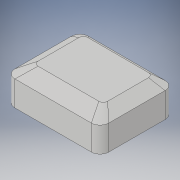
# Autodesk Inventor part: printer
Saved by Autodesk Inventor 2017 (Build 210142000, 142)
## iProperties
Created: 2018-04-03
Part Number: printer
Material: Generic
Document SubType Name: Modeling
Designer: Braxton
Density: 1 g/cm^3
Appearance: Default
Author: Braxton
Autodesk Inventor part; units mm, degrees
ref_plane "YZ Plane" through (0, 0, 0) normal (1, 0, 0) x (0, 1, 0)
ref_plane "XZ Plane" through (0, 0, 0) normal (0, 1, 0) x (-1, 0, 0)
ref_plane "XY Plane" through (0, 0, 0) normal (0, 0, 1) x (1, 0, 0)
sketch "Sketch1" plane through (0, 0, 0) normal (0, 1, 0) x (-1, 0, 0)
  line L0 (20.6375, 12.3693) -> (20.6375, -12.3693)
  line L1 (16.801, 16.2057) -> (0, 16.2057)
  line L2 (0, 0) -> (0, 16.2057) construction
  line L3 (16.801, -16.2057) -> (0, -16.2057)
  arc A0 (16.801, -16.2057) -> (20.6375, -12.3693) centre (16.801, -12.3693) ccw
  arc A1 (20.6375, 12.3693) -> (16.801, 16.2057) centre (16.801, 12.3693) ccw
  line L4 (20.6375, 0) -> (0, 0) construction
  line L5 (-20.6375, 12.3693) -> (-20.6375, -12.3693)
  line L6 (-16.801, 16.2057) -> (0, 16.2057)
  line L7 (-16.801, -16.2057) -> (0, -16.2057)
  arc A2 (-20.6375, -12.3693) -> (-16.801, -16.2057) centre (-16.801, -12.3693) ccw
  arc A3 (-16.801, 16.2057) -> (-20.6375, 12.3693) centre (-16.801, 12.3693) ccw
  line L8 (-20.6375, 0) -> (0, 0) construction
  dimension "d3" = 3.8365
  dimension "d4" = 32.4115
  dimension "d5" = 3.8365
  dimension "d6" = 20.6375
  constraints: 18 end point, 8 point on circle, 7 symmetric about line, 4 centre point, 4 tangent, 3 perpendicular, 1 coincident, 1 horizontal, 1 midpoint, 1 point on line, 2 other
  measures "d3" radius of A0
  measures "d4" distance between parallel lines of L1 L3
  measures "d5" radius of A1
  measures "d6" distance from line of L1.end L0
extrude "middle of body" add sketch "Sketch1" along normal blind 11.0384
ref_plane "top of printer" through (0, 14.2304, 0) normal (0, 1, 0) x (1, 0, 0)
sketch "Sketch2" plane through (0, 14.2304, 0) normal (0, 1, 0) x (1, 0, 0)
  line L0 (-13.3615, -9.4589) -> (0, -9.4589)
  line L1 (0, 12.3693) -> (-13.3615, 12.3693)
  line L2 (-15.2797, 10.451) -> (-15.2797, -7.5406)
  arc A0 (-15.2797, -7.5406) -> (-13.3615, -9.4589) centre (-13.3615, -7.5406) ccw
  arc A1 (-13.3615, 12.3693) -> (-15.2797, 10.451) centre (-13.3615, 10.451) ccw
  line L3 (0, -9.4589) -> (0, 0) construction
  line L4 (0, 0) -> (0, 12.3693) construction
  line L5 (16.801, 16.2057) -> (-16.801, 16.2057) projected
  line L6 (13.3615, -9.4589) -> (0, -9.4589)
  line L7 (0, 12.3693) -> (13.3615, 12.3693)
  line L8 (15.2797, 10.451) -> (15.2797, -7.5406)
  arc A2 (13.3615, -9.4589) -> (15.2797, -7.5406) centre (13.3615, -7.5406) ccw
  arc A3 (15.2797, 10.451) -> (13.3615, 12.3693) centre (13.3615, 10.451) ccw
  dimension "d10" = 15.2797
  dimension "d11" = 21.8281
  dimension "d12" = 3.8365
  dimension "d13" = 1.9182
  constraints: 16 end point, 8 point on circle, 6 symmetric about line, 4 centre point, 4 tangent, 2 perpendicular, 1 coincident, 1 collinear, 1 equal radius, 2 other
  measures "d10" distance from line of L1.start L2
  measures "d11" distance between parallel lines of L0 L1
  measures "d12" distance between parallel lines of L5 L1
  measures "d13" radius of A1
loft "top part of printer" add profiles "Sketch2" section 1 edges at (8.4005, 11.0384, 16.2057) (-8.4005, 11.0384, 16.2057) (19.5138, 11.0384, 15.0821) (20.6375, 11.0384, 0) (19.5138, 11.0384, -15.0821) (-8.4005, 11.0384, -16.2057) (8.4005, 11.0384, -16.2057) (-19.5138, 11.0384, -15.0821) (-20.6375, 11.0384, 0) (-19.5138, 11.0384, 15.0821)
sketch "Sketch39" plane through (-16.801, 11.0384, 16.2057) normal (0, 0.9039427, 0.4276535) x (1, 0, 0)
  circle A0 centre (3.4396, 5.0371) radius 0.4043
  line L0 (3.8689, 2.2071) -> (4.0551, 2.2071)
  line L1 (4.0551, 2.2071) -> (4.0551, 2.0209)
  line L2 (4.0551, 2.0209) -> (3.8689, 2.0209)
  line L3 (3.8688, 2.0209) -> (3.8688, 2.2071)
  arc A1 (3.8689, 2.2071) -> (3.8688, 2.2071) centre (3.8689, 2.2071) ccw
  arc A2 (3.8688, 2.0209) -> (3.8689, 2.0209) centre (3.8689, 2.0209) ccw
  line L4 (3.962, 2.2071) -> (3.962, 2.0209)
  arc A3 (4.0551, 2.2071) -> (4.0551, 2.2071) centre (4.0551, 2.2071) ccw
  arc A4 (4.0551, 2.0209) -> (4.0551, 2.0209) centre (4.0551, 2.0209) ccw
  line L5 (4.0551, 2.2632) -> (3.8689, 2.2632)
  arc A5 (3.8689, 2.2632) -> (3.8128, 2.2071) centre (3.8689, 2.2071) ccw
  line L6 (3.8128, 2.2071) -> (3.8128, 2.0209)
  arc A6 (3.8128, 2.0209) -> (3.8689, 1.9648) centre (3.8689, 2.0209) ccw
  line L7 (3.8689, 1.9648) -> (4.0551, 1.9648)
  arc A7 (4.0551, 1.9648) -> (4.1112, 2.0209) centre (4.0551, 2.0209) ccw
  line L8 (4.1112, 2.0209) -> (4.1112, 2.2071)
  arc A8 (4.1112, 2.2071) -> (4.0551, 2.2632) centre (4.0551, 2.2071) ccw
  circle A9 centre (3.4396, 5.0371) radius 0.4604
  arc A10 (5.1922, 4.9492) -> (4.8493, 4.6063) centre (5.1922, 4.6063) ccw
  arc A11 (4.8493, 1.9753) -> (5.1922, 1.6324) centre (5.1922, 1.9753) ccw
  line L9 (6.5077, 5.735) -> (6.5077, 2.5728) construction
  arc A12 (8.1661, 4.6063) -> (7.8232, 4.9492) centre (7.8232, 4.6063) ccw
  arc A13 (7.8232, 1.6324) -> (8.1661, 1.9753) centre (7.8232, 1.9753) ccw
  line L10 (7.8232, 5.0053) -> (5.1922, 5.0053)
  arc A14 (5.1922, 5.0053) -> (4.7932, 4.6063) centre (5.1922, 4.6063) ccw
  line L11 (4.7932, 4.6063) -> (4.7932, 1.9753)
  arc A15 (4.7932, 1.9753) -> (5.1922, 1.5763) centre (5.1922, 1.9753) ccw
  line L12 (5.1922, 1.5763) -> (7.8232, 1.5763)
  arc A16 (7.8232, 1.5763) -> (8.2222, 1.9753) centre (7.8232, 1.9753) ccw
  line L13 (8.2222, 1.9753) -> (8.2222, 4.6063)
  arc A17 (8.2222, 4.6063) -> (7.8232, 5.0053) centre (7.8232, 4.6063) ccw
  arc A18 (10.4923, 5.9298) -> (10.215, 5.6525) centre (10.4923, 5.6525) ccw
  line L14 (17.5445, 6.4989) -> (17.5445, 1.1088) construction
  arc A19 (10.215, 0.9292) -> (10.4923, 0.6519) centre (10.4923, 0.9292) ccw
  arc A20 (24.874, 5.6525) -> (24.5967, 5.9298) centre (24.5967, 5.6525) ccw
  arc A21 (24.5967, 0.6519) -> (24.874, 0.9292) centre (24.5967, 0.9292) ccw
  line L15 (24.5967, 5.9859) -> (10.4923, 5.9859)
  arc A22 (10.4923, 5.9859) -> (10.1589, 5.6525) centre (10.4923, 5.6525) ccw
  line L16 (10.1589, 5.6525) -> (10.1589, 0.9292)
  arc A23 (10.1589, 0.9292) -> (10.4923, 0.5958) centre (10.4923, 0.9292) ccw
  line L17 (10.4923, 0.5958) -> (24.5967, 0.5958)
  arc A24 (24.5967, 0.5958) -> (24.9301, 0.9292) centre (24.5967, 0.9292) ccw
  arc A25 (24.9301, 5.6525) -> (24.5967, 5.9859) centre (24.5967, 5.6525) ccw
  line L18 (10.8682, 5.5287) -> (15.7881, 5.5287)
  line L19 (15.8708, 5.446) -> (15.8708, 1.7707)
  line L20 (15.7881, 1.688) -> (10.8682, 1.688)
  line L21 (10.7855, 1.7707) -> (10.7855, 5.446)
  arc A26 (10.8682, 5.5287) -> (10.7855, 5.446) centre (10.8682, 5.446) ccw
  arc A27 (10.7855, 1.7707) -> (10.8682, 1.688) centre (10.8682, 1.7707) ccw
  line L22 (13.3281, 5.5287) -> (13.3281, 1.688) construction
  arc A28 (15.8708, 5.446) -> (15.7881, 5.5287) centre (15.7881, 5.446) ccw
  arc A29 (15.7881, 1.688) -> (15.8708, 1.7707) centre (15.7881, 1.7707) ccw
  line L23 (15.7881, 5.5848) -> (10.8682, 5.5848)
  arc A30 (10.8682, 5.5848) -> (10.7294, 5.446) centre (10.8682, 5.446) ccw
  line L24 (10.7294, 5.446) -> (10.7294, 1.7707)
  arc A31 (10.7294, 1.7707) -> (10.8682, 1.6319) centre (10.8682, 1.7707) ccw
  line L25 (10.8682, 1.6319) -> (15.7881, 1.6319)
  arc A32 (15.7881, 1.6319) -> (15.9269, 1.7707) centre (15.7881, 1.7707) ccw
  line L26 (15.9269, 1.7707) -> (15.9269, 5.446)
  arc A33 (15.9269, 5.446) -> (15.7881, 5.5848) centre (15.7881, 5.446) ccw
  line L27 (10.7855, 0.6519) -> (10.7855, 1.1451)
  arc A34 (10.8733, 1.2329) -> (10.7855, 1.1451) centre (10.8733, 1.1451) ccw
  arc A35 (10.8733, 1.289) -> (10.7294, 1.1451) centre (10.8733, 1.1451) ccw
  line L28 (10.7294, 1.1451) -> (10.7294, 0.6519)
  line L29 (15.8708, 1.1451) -> (15.8708, 0.6519)
  arc A36 (15.8708, 1.1451) -> (15.7829, 1.2329) centre (15.7829, 1.1451) ccw
  line L30 (15.9269, 0.6519) -> (15.9269, 1.1451)
  arc A37 (15.9269, 1.1451) -> (15.7829, 1.289) centre (15.7829, 1.1451) ccw
  line L31 (16.4973, 5.9298) -> (18.5494, 5.9298)
  line L32 (18.5494, 5.9298) -> (18.5494, 4.6524)
  line L33 (18.5494, 4.6524) -> (16.4973, 4.6524)
  line L34 (16.4973, 4.6524) -> (16.4973, 5.9298)
  line L35 (16.4973, 4.5963) -> (18.5494, 4.5963)
  line L36 (18.5494, 4.5963) -> (18.5494, 3.3189)
  line L37 (18.5494, 3.3189) -> (16.4973, 3.3189)
  line L38 (16.4973, 3.3189) -> (16.4973, 4.5963)
  line L39 (16.4973, 3.2628) -> (18.5494, 3.2628)
  line L40 (18.5494, 3.2628) -> (18.5494, 1.9854)
  line L41 (18.5494, 1.9854) -> (16.4973, 1.9854)
  line L42 (16.4973, 1.9854) -> (16.4973, 3.2628)
  line L43 (16.4973, 1.9293) -> (18.5494, 1.9293)
  line L44 (18.5494, 1.9293) -> (18.5494, 0.6519)
  line L45 (18.5494, 0.6519) -> (16.4973, 0.6519)
  line L46 (16.4973, 0.6519) -> (16.4973, 1.9293)
  line L47 (18.6055, 5.9298) -> (20.6576, 5.9298)
  line L48 (20.6576, 5.9298) -> (20.6576, 4.6524)
  line L49 (20.6576, 4.6524) -> (18.6055, 4.6524)
  line L50 (18.6055, 4.6524) -> (18.6055, 5.9298)
  line L51 (18.6055, 4.5963) -> (20.6576, 4.5963)
  line L52 (20.6576, 4.5963) -> (20.6576, 3.3189)
  line L53 (20.6576, 3.3189) -> (18.6055, 3.3189)
  line L54 (18.6055, 3.3189) -> (18.6055, 4.5963)
  line L55 (18.6055, 3.2628) -> (20.6576, 3.2628)
  line L56 (20.6576, 3.2628) -> (20.6576, 1.9854)
  line L57 (20.6576, 1.9854) -> (18.6055, 1.9854)
  line L58 (18.6055, 1.9854) -> (18.6055, 3.2628)
  line L59 (18.6055, 1.9293) -> (20.6576, 1.9293)
  line L60 (20.6576, 1.9293) -> (20.6576, 0.6519)
  line L61 (20.6576, 0.6519) -> (18.6055, 0.6519)
  line L62 (18.6055, 0.6519) -> (18.6055, 1.9293)
  line L63 (20.7137, 5.9298) -> (22.7658, 5.9298)
  line L64 (22.7658, 5.9298) -> (22.7658, 4.6524)
  line L65 (22.7658, 4.6524) -> (20.7137, 4.6524)
  line L66 (20.7137, 4.6524) -> (20.7137, 5.9298)
  line L67 (20.7137, 4.5963) -> (22.7658, 4.5963)
  line L68 (22.7658, 4.5963) -> (22.7658, 3.3189)
  line L69 (22.7658, 3.3189) -> (20.7137, 3.3189)
  line L70 (20.7137, 3.3189) -> (20.7137, 4.5963)
  line L71 (20.7137, 3.2628) -> (22.7658, 3.2628)
  line L72 (22.7658, 3.2628) -> (22.7658, 1.9854)
  line L73 (22.7658, 1.9854) -> (20.7137, 1.9854)
  line L74 (20.7137, 1.9854) -> (20.7137, 3.2628)
  line L75 (20.7137, 1.9293) -> (22.7658, 1.9293)
  line L76 (22.7658, 1.9293) -> (22.7658, 0.6519)
  line L77 (22.7658, 0.6519) -> (20.7137, 0.6519)
  line L78 (20.7137, 0.6519) -> (20.7137, 1.9293)
  line L79 (24.874, 4.6524) -> (22.8219, 4.6524)
  line L80 (22.8219, 4.6524) -> (22.8219, 5.9298)
  line L81 (22.8219, 4.5963) -> (24.874, 4.5963)
  line L82 (24.874, 4.5963) -> (24.874, 3.3189)
  line L83 (24.874, 3.3189) -> (22.8219, 3.3189)
  line L84 (22.8219, 3.3189) -> (22.8219, 4.5963)
  line L85 (22.8219, 3.2628) -> (24.874, 3.2628)
  line L86 (24.874, 3.2628) -> (24.874, 1.9854)
  line L87 (24.874, 1.9854) -> (22.8219, 1.9854)
  line L88 (22.8219, 1.9854) -> (22.8219, 3.2628)
  line L89 (22.8219, 1.9293) -> (24.874, 1.9293)
  line L90 (22.8219, 0.6519) -> (22.8219, 1.9293)
  line L91 (25.7461, 5.6668) -> (26.4975, 5.6668)
  line L92 (26.4975, 5.6668) -> (26.4975, 4.9154)
  line L93 (26.4975, 4.9154) -> (25.7461, 4.9154)
  line L94 (25.7461, 4.9154) -> (25.7461, 5.6668)
  line L95 (26.1218, 5.6668) -> (26.1218, 4.9154) construction
  arc A38 (25.7461, 5.6668) -> (25.7461, 5.6668) centre (25.7461, 5.6668) ccw
  arc A39 (25.7461, 4.9154) -> (25.7461, 4.9154) centre (25.7461, 4.9154) ccw
  arc A40 (26.4975, 5.6668) -> (26.4975, 5.6668) centre (26.4975, 5.6668) ccw
  arc A41 (26.4975, 4.9154) -> (26.4975, 4.9154) centre (26.4975, 4.9154) ccw
  line L96 (26.4975, 5.7229) -> (25.7461, 5.7229)
  arc A42 (25.7461, 5.7229) -> (25.69, 5.6668) centre (25.7461, 5.6668) ccw
  line L97 (25.69, 5.6668) -> (25.69, 4.9154)
  arc A43 (25.69, 4.9154) -> (25.7461, 4.8593) centre (25.7461, 4.9154) ccw
  line L98 (25.7461, 4.8593) -> (26.4975, 4.8593)
  arc A44 (26.4975, 4.8593) -> (26.5536, 4.9154) centre (26.4975, 4.9154) ccw
  line L99 (26.5536, 4.9154) -> (26.5536, 5.6668)
  arc A45 (26.5536, 5.6668) -> (26.4975, 5.7229) centre (26.4975, 5.6668) ccw
  line L100 (25.7461, 1.9293) -> (26.4975, 1.9293)
  line L101 (26.4975, 1.9293) -> (26.4975, 1.1779)
  line L102 (26.4975, 1.1779) -> (25.7461, 1.1779)
  line L103 (25.7461, 1.1779) -> (25.7461, 1.9293)
  line L104 (26.1218, 1.9293) -> (26.1218, 1.1779) construction
  arc A46 (25.7461, 1.9293) -> (25.7461, 1.9293) centre (25.7461, 1.9293) ccw
  arc A47 (25.7461, 1.1779) -> (25.7461, 1.1779) centre (25.7461, 1.1779) ccw
  arc A48 (26.4975, 1.9293) -> (26.4975, 1.9293) centre (26.4975, 1.9293) ccw
  arc A49 (26.4975, 1.1779) -> (26.4975, 1.1779) centre (26.4975, 1.1779) ccw
  line L105 (26.4975, 1.9854) -> (25.7461, 1.9854)
  arc A50 (25.7461, 1.9854) -> (25.69, 1.9293) centre (25.7461, 1.9293) ccw
  line L106 (25.69, 1.9293) -> (25.69, 1.1779)
  arc A51 (25.69, 1.1779) -> (25.7461, 1.1218) centre (25.7461, 1.1779) ccw
  line L107 (25.7461, 1.1218) -> (26.4975, 1.1218)
  arc A52 (26.4975, 1.1218) -> (26.5536, 1.1779) centre (26.4975, 1.1779) ccw
  line L108 (26.5536, 1.1779) -> (26.5536, 1.9293)
  arc A53 (26.5536, 1.9293) -> (26.4975, 1.9854) centre (26.4975, 1.9293) ccw
  line L109 (25.7461, 3.6665) -> (26.4975, 3.6665)
  line L110 (26.4975, 3.6665) -> (26.4975, 2.9151)
  line L111 (26.4975, 2.9151) -> (25.7461, 2.9151)
  line L112 (25.7461, 2.9151) -> (25.7461, 3.6665)
  line L113 (26.1218, 3.6665) -> (26.1218, 2.9151) construction
  arc A54 (25.7461, 3.6665) -> (25.7461, 3.6665) centre (25.7461, 3.6665) ccw
  arc A55 (25.7461, 2.9151) -> (25.7461, 2.9151) centre (25.7461, 2.9151) ccw
  arc A56 (26.4975, 3.6665) -> (26.4975, 3.6665) centre (26.4975, 3.6665) ccw
  arc A57 (26.4975, 2.9151) -> (26.4975, 2.9151) centre (26.4975, 2.9151) ccw
  line L114 (26.4975, 3.7226) -> (25.7461, 3.7226)
  arc A58 (25.7461, 3.7226) -> (25.69, 3.6665) centre (25.7461, 3.6665) ccw
  line L115 (25.69, 3.6665) -> (25.69, 2.9151)
  arc A59 (25.69, 2.9151) -> (25.7461, 2.859) centre (25.7461, 2.9151) ccw
  line L116 (25.7461, 2.859) -> (26.4975, 2.859)
  arc A60 (26.4975, 2.859) -> (26.5536, 2.9151) centre (26.4975, 2.9151) ccw
  line L117 (26.5536, 2.9151) -> (26.5536, 3.6665)
  arc A61 (26.5536, 3.6665) -> (26.4975, 3.7226) centre (26.4975, 3.6665) ccw
  arc A62 (27.3029, 1.1779) -> (27.359, 1.1218) centre (27.359, 1.1779) ccw
  arc A63 (27.359, 1.1779) -> (27.359, 1.1779) centre (27.359, 1.1779) ccw
  arc A64 (28.9306, 1.1779) -> (28.9306, 1.1779) centre (28.9306, 1.1779) ccw
  arc A65 (28.9306, 1.1218) -> (28.9867, 1.1779) centre (28.9306, 1.1779) ccw
  line L118 (27.359, 1.1218) -> (28.9306, 1.1218)
  line L119 (28.9306, 1.1779) -> (27.359, 1.1779)
  line L120 (27.359, 1.1779) -> (27.359, 2.7495)
  line L121 (27.3029, 2.7495) -> (27.3029, 1.1779)
  arc A66 (27.359, 2.8056) -> (27.3029, 2.7495) centre (27.359, 2.7495) ccw
  arc A67 (27.359, 2.7495) -> (27.359, 2.7495) centre (27.359, 2.7495) ccw
  line L122 (28.1448, 2.7495) -> (28.1448, 1.1779) construction
  line L123 (28.9306, 2.7495) -> (28.9306, 1.1779)
  line L124 (28.9867, 1.1779) -> (28.9867, 2.7495)
  line L125 (27.359, 2.7495) -> (28.9306, 2.7495)
  line L126 (28.9306, 2.8056) -> (27.359, 2.8056)
  arc A68 (28.9306, 2.7495) -> (28.9306, 2.7495) centre (28.9306, 2.7495) ccw
  arc A69 (28.9867, 2.7495) -> (28.9306, 2.8056) centre (28.9306, 2.7495) ccw
  arc A70 (27.3029, 4.0952) -> (27.359, 4.0391) centre (27.359, 4.0952) ccw
  arc A71 (27.359, 4.0952) -> (27.359, 4.0952) centre (27.359, 4.0952) ccw
  arc A72 (28.9306, 4.0952) -> (28.9306, 4.0952) centre (28.9306, 4.0952) ccw
  arc A73 (28.9306, 4.0391) -> (28.9867, 4.0952) centre (28.9306, 4.0952) ccw
  line L127 (27.359, 4.0391) -> (28.9306, 4.0391)
  line L128 (28.9306, 4.0952) -> (27.359, 4.0952)
  line L129 (27.359, 4.0952) -> (27.359, 5.6668)
  line L130 (27.3029, 5.6668) -> (27.3029, 4.0952)
  arc A74 (27.359, 5.7229) -> (27.3029, 5.6668) centre (27.359, 5.6668) ccw
  arc A75 (27.359, 5.6668) -> (27.359, 5.6668) centre (27.359, 5.6668) ccw
  line L131 (28.1448, 5.6668) -> (28.1448, 4.0952) construction
  line L132 (28.9306, 5.6668) -> (28.9306, 4.0952)
  line L133 (28.9867, 4.0952) -> (28.9867, 5.6668)
  line L134 (27.359, 5.6668) -> (28.9306, 5.6668)
  line L135 (28.9306, 5.7229) -> (27.359, 5.7229)
  arc A76 (28.9306, 5.6668) -> (28.9306, 5.6668) centre (28.9306, 5.6668) ccw
  arc A77 (28.9867, 5.6668) -> (28.9306, 5.7229) centre (28.9306, 5.6668) ccw
  circle A78 centre (30.3038, 5.2599) radius 0.4069
  circle A79 centre (30.3038, 5.2599) radius 0.463
  line L136 (30.6845, 1.1779) -> (30.2692, 1.1779)
  line L137 (30.12, 1.4364) -> (30.3276, 1.796)
  line L138 (30.6261, 1.796) -> (30.8337, 1.4364)
  arc A80 (30.6261, 1.796) -> (30.3276, 1.796) centre (30.4768, 1.7098) ccw
  arc A81 (30.12, 1.4364) -> (30.2692, 1.1779) centre (30.2692, 1.3502) ccw
  arc A82 (30.6845, 1.1779) -> (30.8337, 1.4364) centre (30.6845, 1.3502) ccw
  line L139 (30.279, 1.824) -> (30.0714, 1.4644)
  arc A83 (30.0714, 1.4644) -> (30.2692, 1.1218) centre (30.2692, 1.3502) ccw
  line L140 (30.2692, 1.1218) -> (30.6845, 1.1218)
  arc A84 (30.6845, 1.1218) -> (30.8823, 1.4644) centre (30.6845, 1.3502) ccw
  line L141 (30.8823, 1.4644) -> (30.6747, 1.824)
  arc A85 (30.6747, 1.824) -> (30.279, 1.824) centre (30.4768, 1.7098) ccw
  line L142 (6.5077, 5.735) -> (6.5077, 5.0053) construction
  line L143 (4.8493, 3.3189) -> (6.4796, 3.3189)
  line L144 (6.5357, 3.3189) -> (8.1661, 3.3189)
  line L145 (8.1661, 3.2628) -> (6.5357, 3.2628)
  line L146 (6.4796, 3.2628) -> (4.8493, 3.2628)
  line L147 (6.4796, 1.6324) -> (6.4796, 3.2628)
  line L148 (6.4796, 3.3189) -> (6.4796, 4.9492)
  line L149 (6.5357, 4.9492) -> (6.5357, 3.3189)
  line L150 (6.5357, 3.2628) -> (6.5357, 1.6324)
  line L151 (8.1661, 4.6063) -> (8.1661, 3.3189)
  line L152 (8.1661, 3.2628) -> (8.1661, 1.9753)
  line L153 (7.8232, 1.6324) -> (6.5357, 1.6324)
  line L154 (6.4796, 1.6324) -> (5.1922, 1.6324)
  line L155 (4.8493, 1.9753) -> (4.8493, 3.2628)
  line L156 (4.8493, 3.3189) -> (4.8493, 4.6063)
  line L157 (5.1922, 4.9492) -> (6.4796, 4.9492)
  line L158 (6.5357, 4.9492) -> (7.8232, 4.9492)
  line L159 (10.215, 0.9292) -> (10.215, 5.6525)
  line L160 (30.1625, 7.4638) -> (3.4396, 7.4638) projected
  line L161 (3.4396, 7.4638) -> (3.4396, 5.0371) construction
  line L162 (4.7932, 3.2908) -> (8.2222, 3.2908) construction
  line L163 (10.8733, 1.289) -> (15.7829, 1.289)
  line L164 (22.8219, 5.9298) -> (24.5967, 5.9298)
  line L165 (24.874, 5.6525) -> (24.874, 4.6524)
  line L166 (24.874, 1.9293) -> (24.874, 0.9292)
  line L167 (24.5967, 0.6519) -> (22.8219, 0.6519)
  line L168 (24.9301, 5.6525) -> (24.9301, 0.9292)
  line L169 (3.4396, 5.0371) -> (3.9, 5.0371) construction
  line L170 (10.4923, 5.9298) -> (16.4412, 5.9298)
  line L171 (16.4412, 5.9298) -> (16.4412, 0.6519)
  line L172 (10.4923, 0.6519) -> (10.7294, 0.6519)
  line L173 (15.9269, 0.6519) -> (16.4412, 0.6519)
  line L174 (12.4261, 1.2329) -> (12.4261, 0.6519)
  line L175 (12.5351, 0.6519) -> (12.5351, 1.2329)
  line L176 (14.1212, 1.2329) -> (14.1212, 0.6519)
  line L177 (14.2302, 0.6519) -> (14.2302, 1.2329)
  line L178 (12.37, 1.2329) -> (12.37, 0.6519)
  line L179 (12.5912, 1.2329) -> (12.5912, 0.6519)
  line L180 (14.0651, 1.2329) -> (14.0651, 0.6519)
  line L181 (14.2863, 1.2329) -> (14.2863, 0.6519)
  line L182 (10.8733, 1.2329) -> (12.37, 1.2329)
  line L183 (10.7855, 0.6519) -> (12.37, 0.6519)
  line L184 (12.4261, 0.6519) -> (12.5351, 0.6519)
  line L185 (12.4261, 1.2329) -> (12.5351, 1.2329)
  line L186 (12.5912, 1.2329) -> (14.0651, 1.2329)
  line L187 (12.5912, 0.6519) -> (14.0651, 0.6519)
  line L188 (14.1212, 0.6519) -> (14.2302, 0.6519)
  line L189 (14.2863, 0.6519) -> (15.8708, 0.6519)
  line L190 (14.1212, 1.2329) -> (14.2302, 1.2329)
  line L191 (14.2863, 1.2329) -> (15.7829, 1.2329)
  line L192 (10.1589, 3.2908) -> (8.2222, 3.2908) construction
  line L193 (30.3038, 5.2599) -> (30.3038, 5.7229) construction
  line L194 (30.3038, 5.7229) -> (29.3869, 5.7229) construction
  line L195 (25.7461, 5.2911) -> (26.4975, 5.2911) construction
  line L196 (22.8219, 5.2911) -> (24.874, 5.2911) construction
  line L197 (24.9301, 3.2908) -> (25.2661, 3.2908) construction
  line L198 (25.7461, 3.2908) -> (26.4975, 3.2908) construction
  line L199 (30.6845, 1.3502) -> (30.6257, 1.3502) construction
  line L200 (29.8408, 5.2599) -> (30.3038, 5.2599) construction
  point P0 (16.801, 9.9284)
  point P1 (30.4768, 1.4701)
  point P2 (3.4396, 5.4974)
  point P3 (12.4806, 1.2329)
  point P4 (14.1757, 1.2329)
  point P5 (30.0408, 1.3502)
  dimension "d226" = 0.0561
  dimension "d227" = 0.0561
  dimension "d232" = 0.0561
  dimension "d236" = 0.0561
  dimension "d238" = 0.0561
  dimension "d243" = 0.0561
  dimension "d244" = 0.0561
  dimension "d245" = 0.0561
  dimension "d246" = 0.0561
  dimension "d247" = 0.0561
  dimension "d248" = 0.0561
  dimension "d251" = 360
  dimension "d253" = 0.0561
  dimension "d274" = 0.8086
  dimension "d275" = 0.1863
  dimension "d276" = 0.0561
  dimension "d278" = 0.028
  dimension "d279" = 0.0561
  dimension "d280" = 0.0561
  dimension "d281" = 0.0561
  dimension "d282" = 0.0561
  dimension "d283" = 0.0561
  dimension "d284" = 3.3168
  dimension "d285" = 3.3168
  dimension "d286" = 0.0561
  dimension "d287" = 0.0561
  dimension "d288" = 5.0853
  dimension "d289" = 3.8407
  dimension "d290" = 0.0561
  dimension "d291" = 0.0561
  dimension "d292" = 0.0561
  dimension "d293" = 0.0561
  dimension "d294" = 0.0561
  dimension "d295" = 0.0561
  dimension "d297" = 0.4932
  dimension "d298" = 0.0878
  dimension "d300" = 0.3429
  dimension "d301" = 1.2774
  dimension "d302" = 2.0521
  dimension "d305" = 1.9664
  dimension "d306" = 0.8932
  dimension "d308" = 2.4585
  dimension "d309" = 0.2773
  dimension "d310" = 0.0561
  dimension "d311" = 0.109
  dimension "d312" = 0.109
  dimension "d313" = 0.0561
  dimension "d314" = 0.0561
  dimension "d315" = 0.0561
  dimension "d316" = 0.0561
  dimension "d317" = 1.6951
  dimension "d318" = 1.6951
  dimension "d319" = 0.3429
  dimension "d320" = 1.9928
  dimension "d321" = 0.5143
  dimension "d322" = 0.5143
  dimension "d323" = 0.0561
  dimension "d324" = 0.7514
  dimension "d325" = 1.5716
  dimension "d327" = 0.7599
  dimension "d328" = 0.7493
  dimension "d329" = 0.8139
  dimension "d331" = 1.0541
  dimension "d332" = 0.8541
  constraints: 395 end point, 169 point on circle, 86 centre point, 79 parallel, 69 perpendicular, 62 tangent, 60 collinear, 54 symmetric about line, 42 horizontal, 27 equal length, 26 midpoint, 14 equal radius, 3 point on line, 3 vertical, 104 other
  measures "d226" distance between parallel lines of L0 L5
  measures "d227" radial gap between concentric circles of A0 A9
  measures "d232" distance between parallel lines of L18 L23
  measures "d236" radial gap between concentric circles of A22 A18
  measures "d238" radial gap between concentric circles of A25 A20
  measures "d243" distance between parallel lines of L91 L96
  measures "d244" distance between parallel lines of L100 L105
  measures "d245" distance between parallel lines of L109 L114
  measures "d246" distance between parallel lines of L125 L126
  measures "d247" distance between parallel lines of L134 L135
  measures "d248" radial gap between concentric circles of A78 A79
  measures "d253" distance between parallel lines of L137 L139
  measures "d274" diameter of A0
  measures "d275" distance between parallel lines of L1 L3
  measures "d276" distance between parallel lines of L10 L157
  measures "d278" distance between parallel lines of L143 L162
  measures "d279" distance between parallel lines of L146 L143
  measures "d280" radial gap between concentric circles of A10 A14
  measures "d281" distance between parallel lines of L156 L11
  measures "d282" radial gap between concentric circles of A15 A11
  measures "d284" distance between parallel lines of L154 L157
  measures "d285" distance between parallel lines of L151 L156
  measures "d286" diameter of L148 L9
  measures "d287" distance between parallel lines of L149 L148
  measures "d288" distance between parallel lines of L19 L21
  measures "d289" distance between parallel lines of L18 L20
  measures "d290" distance between parallel lines of L35 L33
  measures "d291" distance between parallel lines of L37 L39
  measures "d292" distance between parallel lines of L41 L43
  measures "d293" distance between parallel lines of L50 L32
  measures "d294" distance between parallel lines of L48 L66
  measures "d295" distance between parallel lines of L64 L80
  measures "d297" distance of L27.start L27.end
  measures "d298" radius of A34
  measures "d300" distance between parallel lines of L25 L163
  measures "d301" distance of L33.end L31.start
  measures "d302" distance of L31.start L31.end
  measures "d305" distance of L160.end A9.start
  measures "d306" distance from line of L11 L169.end
  measures "d308" distance between parallel lines of L160 L10
  measures "d309" radius of A18
  measures "d310" distance between parallel lines of L34 L171
  measures "d311" distance between parallel lines of L175 L174
  measures "d312" distance between parallel lines of L177 L176
  measures "d313" distance between parallel lines of L174 L178
  measures "d314" distance between parallel lines of L179 L175
  measures "d315" distance between parallel lines of L176 L180
  measures "d316" distance between parallel lines of L181 L177
  measures "d317" distance from line of L27 point (12.481, 1.233)
  measures "d318" distance of point (14.176, 1.233) point (12.481, 1.233)
  measures "d319" radius of A10
  measures "d320" distance between parallel lines of L13 L159
  measures "d321" distance between parallel lines of L159 L24
  measures "d322" distance between parallel lines of L171 L26
  measures "d323" radial gap between concentric circles of A35 A34
  measures "d324" distance between parallel lines of L94 L92
  measures "d325" distance between parallel lines of L123 L120
  measures "d327" distance between parallel lines of L97 L168
  measures "d328" distance between parallel lines of L130 L99
  measures "d329" diameter of A78
  measures "d331" distance from line of L124 point (30.041, 1.35)
  measures "d332" distance from line of L133 L200.start
extrude "keys for printer" [suppressed]
sketch "Sketch3" plane through (0, -4.5328, 0) normal (0, -1, 0) x (1, 0, 0)
  line L0 (16.801, -16.2057) -> (-16.801, -16.2057) projected
  line L1 (-18.124, -15.9704) -> (-18.124, 11.5314)
  line L2 (-15.5663, 14.0891) -> (0, 14.0891)
  line L3 (0, 14.0891) -> (0, -16.2057) construction
  arc A0 (-15.5663, 14.0891) -> (-18.124, 11.5314) centre (-15.5663, 11.5314) ccw
  line L4 (-16.801, 16.2057) -> (16.801, 16.2057) projected
  line L5 (-16.801, -16.2057) -> (0, -16.2057)
  line L6 (18.124, -15.9704) -> (18.124, 11.5314)
  line L7 (15.5663, 14.0891) -> (0, 14.0891)
  arc A1 (18.124, 11.5314) -> (15.5663, 14.0891) centre (15.5663, 11.5314) ccw
  line L8 (16.801, -16.2057) -> (0, -16.2057)
  line L9 (16.801, -16.2057) -> (-16.801, -16.2057) projected
  arc A2 (16.801, -16.2057) -> (20.6375, -12.3693) centre (16.801, -12.3693) ccw projected
  arc A3 (16.801, -16.2057) -> (18.124, -15.9704) centre (16.801, -12.3693) ccw
  arc A4 (-20.6375, -12.3693) -> (-16.801, -16.2057) centre (-16.801, -12.3693) ccw projected
  arc A5 (-18.124, -15.9704) -> (-16.801, -16.2057) centre (-16.801, -12.3693) ccw
  point P0 (0, 0)
  dimension "d19" = 18.124
  dimension "d21" = 2.1167
  dimension "d22" = 2.5576
  constraints: 14 end point, 12 point on circle, 4 centre point, 3 symmetric about line, 3 tangent, 3 vertical, 2 concentric, 1 midpoint, 1 perpendicular, 1 other
  measures "d19" distance from line of L2.end L1
  measures "d21" distance between parallel lines of L4 L2
  measures "d22" radius of A0
sketch "Sketch7" plane through (0, 0, 0) normal (0, 1, 0) x (-1, 0, 0)
  line L0 (17.2445, 14.6352) -> (0, 14.6352)
  arc A0 (18.9061, 14.3929) -> (17.2445, 14.6352) centre (17.2445, 8.8168) ccw
  line L1 (0, 14.6352) -> (0, 0) construction
  line L2 (16.801, 16.2057) -> (-16.801, 16.2057) projected
  line L3 (20.6375, -12.3693) -> (20.6375, 12.3693) projected
  line L4 (18.9061, 14.3929) -> (19.5668, 15.028)
  arc A1 (20.6375, 12.3693) -> (16.801, 16.2057) centre (16.801, 12.3693) ccw projected
  arc A2 (19.5668, 15.028) -> (16.801, 16.2057) centre (16.801, 12.3693) ccw
  line L5 (16.801, 16.2057) -> (13.3615, 9.4589) projected
  line L6 (16.801, 16.2057) -> (0, 16.2057)
  line L7 (-17.2445, 14.6352) -> (0, 14.6352)
  arc A3 (-17.2445, 14.6352) -> (-18.9061, 14.3929) centre (-17.2445, 8.8168) ccw
  line L8 (-18.9061, 14.3929) -> (-19.5668, 15.028)
  arc A4 (-16.801, 16.2057) -> (-19.5668, 15.028) centre (-16.801, 12.3693) ccw
  line L9 (-16.801, 16.2057) -> (0, 16.2057)
  point P0 (-16.801, 12.3693)
  dimension "d43" = 1.5706
  dimension "d46" = 0.4434
  dimension "d47" = 0.9165
  dimension "d48" = 1.7314
  dimension "d87" = 33.6021
  constraints: 14 end point, 9 point on circle, 6 symmetric about line, 4 centre point, 1 concentric, 1 horizontal, 1 line through centre, 1 midpoint, 1 tangent, 1 vertical, 2 other
  measures "d43" distance between parallel lines of L2 L0
  measures "d46" horizontal distance of L0.start L2.start
  measures "d47" distance of L4.start L4.end
  measures "d48" distance from line of L3 L4.start
  measures "d87" distance of L2.end L2.start
sketch "Sketch9" plane through (0, 6.4537, 0) normal (0, -1, 0) x (1, 0, 0)
  line L0 (-16.801, 16.2057) -> (16.801, 16.2057) projected
  line L1 (0, 16.2057) -> (-16.801, 16.2057)
  arc A0 (-19.5668, 15.028) -> (-20.6375, 12.3693) centre (-16.801, 12.3693) ccw projected
  arc A1 (-16.801, 16.2057) -> (-20.1955, 14.1569) centre (-16.801, 12.3693) ccw
  line L2 (0, 15.7443) -> (-15.5183, 15.7443)
  line L3 (0, 16.2057) -> (0, 15.7443) construction
  line L4 (17.2445, 14.6352) -> (-17.2445, 14.6352) projected
  line L5 (-20.6375, -12.3693) -> (-20.6375, 12.3693) projected
  line L6 (-20.1955, 14.1569) -> (-19.8772, 13.9893)
  arc A2 (-15.5183, 15.7443) -> (-18.9061, 14.3929) centre (-15.5183, 10.8225) ccw
  line L7 (-18.9061, 14.3929) -> (-19.8772, 13.9893)
  line L8 (0, 16.2057) -> (16.801, 16.2057)
  arc A3 (20.1955, 14.1569) -> (16.801, 16.2057) centre (16.801, 12.3693) ccw
  line L9 (0, 15.7443) -> (15.5183, 15.7443)
  line L10 (20.1955, 14.1569) -> (19.8772, 13.9893)
  arc A4 (18.9061, 14.3929) -> (15.5183, 15.7443) centre (15.5183, 10.8225) ccw
  line L11 (18.9061, 14.3929) -> (19.8772, 13.9893)
  point P0 (0, 0)
  point P1 (19.5668, 15.028)
  point P2 (16.801, 12.3693)
  dimension "d57" = 1.1091
  dimension "d62" = 0.3598
  dimension "d63" = 1.8415
  dimension "d64" = 1.2827
  constraints: 18 end point, 9 point on circle, 8 symmetric about line, 4 centre point, 1 collinear, 1 concentric, 1 horizontal, 1 line through centre, 1 midpoint, 1 perpendicular, 1 tangent, 2 other
  measures "d57" distance between parallel lines of L4 L2
  measures "d62" distance of L6.start L6.end
  measures "d63" distance of L6.start L5.end
  measures "d64" horizontal distance of L2.end L0.start
sketch "Sketch4" plane through (16.801, 11.0384, -16.2057) normal (0, 0, -1) x (-1, 0, 0)
  line L0 (37.4385, -15.5713) -> (37.4385, -5.8028)
  line L1 (37.4385, -11.0384) -> (37.4385, 0) projected
  line L2 (37.4385, -5.8028) -> (34.0117, -5.8028)
  line L3 (33.6137, -6.2008) -> (33.6137, -7.3745)
  line L4 (33.6021, -15.5713) -> (0, -15.5713) projected
  line L5 (37.4385, -15.5713) -> (28.0617, -15.5713)
  line L6 (28.0617, -15.5713) -> (28.0617, -9.4435)
  line L7 (29.5857, -7.9195) -> (33.0687, -7.9195)
  arc A0 (29.5857, -7.9195) -> (28.0617, -9.4435) centre (29.5857, -9.4435) ccw
  arc A1 (33.0687, -7.9195) -> (33.6137, -7.3745) centre (33.0687, -7.3745) ccw
  arc A2 (34.0117, -5.8028) -> (33.6137, -6.2008) centre (34.0117, -6.2008) ccw
  point P0 (16.801, -11.0384)
  dimension "d27" = 9.7684
  dimension "d30" = 9.3768
  dimension "d33" = 2.1167
  dimension "d36" = 1.524
  dimension "d37" = 0.545
  dimension "d38" = 0.3979
  dimension "d39" = 3.8248
  constraints: 12 end point, 6 point on circle, 6 tangent, 3 centre point, 3 vertical, 2 point on line, 1 collinear, 1 horizontal, 1 perpendicular
  measures "d27" distance of L0.start L0.end
  measures "d30" distance of L0.start L5.end
  measures "d33" distance between parallel lines of L2 L7
  measures "d36" radius of A0
  measures "d37" radius of A1
  measures "d38" radius of A2
  measures "d39" distance between parallel lines of L0 L3
sketch "Sketch5" plane through (-16.8127, 3.664, -16.2057) normal (-1, 0, 0) x (0, 0, 1)
  arc A0 (2.94, 0.3503) -> (1.7187, 1.5716) centre (1.7187, 0.3503) ccw
  line L0 (2.94, 1.5716) -> (0.0219, 1.5716) projected
  line L1 (2.94, 1.5716) -> (0, 1.5716)
  line L2 (2.94, 0.3503) -> (2.94, 1.5716)
  line L3 (2.94, 1.5716) -> (1.7187, 1.5716)
  point P0 (16.2057, -3.664)
  dimension "d40" = 1.2213
  constraints: 6 end point, 2 point on circle, 2 tangent, 1 centre point, 1 horizontal, 1 perpendicular, 1 vertical
  measures "d40" radius of A0
sketch "Sketch21" plane through (-17.2445, 0, 14.6352) normal (0, 0, 1) x (1, 0, 0)
  line L0 (0.4434, 0) -> (34.0455, 0) projected
  line L1 (17.2445, 0) -> (26.8356, 0)
  line L2 (26.8356, 0) -> (26.8356, 2.2659)
  line L3 (26.8356, 2.2659) -> (17.2445, 2.2659)
  line L4 (17.2445, 2.2659) -> (17.2445, 0) construction
  line L5 (17.2445, 0) -> (7.6533, 0)
  line L6 (7.6533, 0) -> (7.6533, 2.2659)
  line L7 (7.6533, 2.2659) -> (17.2445, 2.2659)
  dimension "d116" = 9.5912
  dimension "d117" = 2.2659
  constraints: 14 end point, 3 perpendicular, 2 symmetric about line, 1 midpoint, 1 point on line
  measures "d116" distance of L1.start L1.end
  measures "d117" distance of L1.end L2.end
sketch "Sketch22" plane through (-17.2445, 0, 9.4821) normal (0, 0, 1) x (1, 0, 0)
  line L0 (26.8356, 0) -> (7.6533, 0) projected
  line L1 (7.6533, 0) -> (7.6533, 2.2659) projected
  line L2 (7.6533, 0) -> (7.6533, 2.2659)
  line L3 (7.6533, 2.2659) -> (26.8356, 2.2659) projected
  line L4 (7.6533, 2.2659) -> (26.8356, 2.2659)
  line L5 (26.8356, 2.2659) -> (26.8356, 0) projected
  line L6 (26.8356, 2.2659) -> (26.8356, 0)
  line L7 (26.8356, 0) -> (7.6533, 0)
  point P0 (17.2445, 0)
  constraints: 8 end point, 2 collinear, 2 perpendicular
sketch "Sketch23" plane through (-17.2445, 6.4537, 14.6352) normal (0, 0, 1) x (1, 0, 0)
  line L0 (34.489, 0) -> (0, 0) projected
  line L1 (17.2445, 0) -> (24.8983, 0)
  line L2 (24.8983, 0) -> (24.8983, -1.7928)
  line L3 (24.8983, -1.7928) -> (17.2445, -1.7928)
  line L4 (17.2445, -1.7928) -> (17.2445, 0) construction
  line L5 (17.2445, 0) -> (9.5906, 0)
  line L6 (9.5906, 0) -> (9.5906, -1.7928)
  line L7 (9.5906, -1.7928) -> (17.2445, -1.7928)
  point P0 (17.2445, -6.4537)
  dimension "d121" = 7.6539
  dimension "d122" = 1.7928
  constraints: 14 end point, 2 perpendicular, 2 symmetric about line, 1 midpoint, 1 point on line, 1 vertical
  measures "d121" distance of L1.start L1.end
  measures "d122" distance of L1.end L2.end
sketch "Sketch24" plane through (-17.2445, 0, 14.6352) normal (0, 0, 1) x (1, 0, 0)
  line L0 (24.8983, 4.6609) -> (9.5906, 4.6609) projected
  line L1 (17.2445, 4.6609) -> (17.2445, 3.8312) construction
  line L2 (17.2445, 3.8312) -> (19.1685, 3.8312)
  line L3 (19.1685, 3.8312) -> (19.1685, 4.6609)
  line L4 (17.2445, 4.6609) -> (19.1685, 4.6609)
  line L5 (17.2445, 3.8312) -> (15.3204, 3.8312)
  line L6 (15.3204, 3.8312) -> (15.3204, 4.6609)
  line L7 (17.2445, 4.6609) -> (15.3204, 4.6609)
  point P0 (17.2445, 0)
  dimension "d125" = 0.8297
  dimension "d126" = 1.9241
  constraints: 14 end point, 3 perpendicular, 2 symmetric about line, 1 midpoint, 1 point on line, 1 vertical
  measures "d125" distance of L1.start L1.end
  measures "d126" distance of L1.end L2.end
sketch "Sketch25" plane through (-16.801, 11.0384, 16.2057) normal (0, 0, 1) x (1, 0, 0)
  line L0 (32.3194, -1.0192) -> (1.2827, -1.0192) projected
  line L1 (16.801, -1.0192) -> (16.801, 0) construction
  line L2 (33.6021, 0) -> (0, 0) projected
  line L3 (16.801, 0) -> (21.0344, 0)
  line L4 (21.0344, 0) -> (21.0344, -1.0192)
  line L5 (16.801, -1.0192) -> (21.0344, -1.0192)
  line L6 (16.801, 0) -> (12.5677, 0)
  line L7 (12.5677, 0) -> (12.5677, -1.0192)
  line L8 (16.801, -1.0192) -> (12.5677, -1.0192)
  point P0 (16.801, -11.0384)
  dimension "d129" = 4.2333
  constraints: 14 end point, 2 midpoint, 2 perpendicular, 2 symmetric about line, 1 collinear, 1 point on line
  measures "d129" distance of L1.end L3.end
sketch "Sketch35" plane through (16.801, 10.0192, 16.2057) normal (0, 0, 1) x (1, 0, 0)
  line L0 (-20.729, -11.5729) -> (-16.801, -11.5729)
  line L1 (-16.801, -13.1286) -> (-20.729, -13.1286)
  line L2 (-21.0344, -12.8232) -> (-21.0344, -11.8783)
  line L3 (-16.801, -11.5729) -> (-16.801, -13.1286) construction
  line L4 (-16.801, -10.0192) -> (-16.801, -10.8163) construction
  arc A0 (-20.729, -11.5729) -> (-21.0344, -11.8783) centre (-20.729, -11.8783) ccw
  arc A1 (-21.0344, -12.8232) -> (-20.729, -13.1286) centre (-20.729, -12.8232) ccw
  line L5 (-12.8731, -11.5729) -> (-16.801, -11.5729)
  line L6 (-16.801, -13.1286) -> (-12.8731, -13.1286)
  line L7 (-12.5677, -12.8232) -> (-12.5677, -11.8783)
  arc A2 (-12.5677, -11.8783) -> (-12.8731, -11.5729) centre (-12.8731, -11.8783) ccw
  arc A3 (-12.8731, -13.1286) -> (-12.5677, -12.8232) centre (-12.8731, -12.8232) ccw
  line L8 (-33.6021, -10.0192) -> (0, -10.0192) projected
  point P0 (-17.2445, -16.876)
  dimension "d201" = 1.5557
  dimension "d202" = 1.5536
  dimension "d203" = 0.3054
  dimension "d204" = 8.4667
  constraints: 16 end point, 8 point on circle, 6 symmetric about line, 4 centre point, 4 tangent, 1 collinear, 1 equal radius, 1 horizontal, 1 midpoint, 1 parallel, 1 vertical, 2 other
  measures "d201" distance between parallel lines of L0 L1
  measures "d202" distance from line of L4.start L0
  measures "d203" radius of A0
  measures "d204" diameter of L2 L3
sketch "Sketch37" plane through (-15.5663, -4.5328, 14.0891) normal (0, -0.4231055, 0.9060804) x (1, 0, 0)
  line L0 (31.1326, 0) -> (0, 0) projected
  line L1 (-1.2347, 5.0027) -> (32.3674, 5.0027) projected
  line L2 (3.0674, 5.0027) -> (3.2198, 5.0027)
  line L3 (3.2198, 5.0027) -> (3.2198, 2.6741)
  line L4 (3.0674, 2.5217) -> (3.0674, 5.0027)
  line L5 (11.333, 2.5217) -> (11.333, 2.6741)
  line L6 (11.333, 2.6741) -> (3.2198, 2.6741)
  line L7 (4.4274, 2.5217) -> (4.4274, 0)
  line L8 (4.4274, 0) -> (4.275, 0)
  line L9 (4.275, 0) -> (4.275, 2.5217)
  line L10 (3.0674, 2.5217) -> (4.275, 2.5217)
  line L11 (4.4274, 2.5217) -> (11.333, 2.5217)
  line L12 (11.333, 1.9081) -> (11.333, 2.9509) projected
  line L13 (15.5663, 5.0027) -> (15.5663, 0)
  line L14 (28.0652, 5.0027) -> (27.9128, 5.0027)
  line L15 (27.9128, 5.0027) -> (27.9128, 2.6741)
  line L16 (28.0652, 2.5217) -> (28.0652, 5.0027)
  line L17 (19.7997, 2.5217) -> (19.7997, 2.6741)
  line L18 (19.7997, 2.6741) -> (27.9128, 2.6741)
  line L19 (26.7053, 2.5217) -> (26.7053, 0)
  line L20 (26.7053, 0) -> (26.8577, 0)
  line L21 (26.8577, 0) -> (26.8577, 2.5217)
  line L22 (28.0652, 2.5217) -> (26.8577, 2.5217)
  line L23 (26.7053, 2.5217) -> (19.7997, 2.5217)
  line L24 (19.7997, 1.9081) -> (19.7997, 2.9509)
  point P0 (15.5663, -1.854)
  dimension "d218" = 0.1524
  dimension "d219" = 0.1524
  dimension "d220" = 0.1524
  dimension "d223" = 8.2656
  dimension "d224" = 6.9056
  constraints: 44 end point, 12 symmetric about line, 5 perpendicular, 4 parallel, 4 point on line, 3 horizontal, 2 midpoint, 1 collinear
  measures "d218" distance between parallel lines of L3 L4
  measures "d219" distance between parallel lines of L6 L10
  measures "d220" distance between parallel lines of L9 L7
  measures "d223" distance between parallel lines of L5 L4
  measures "d224" distance between parallel lines of L5 L7
sketch "Sketch15" plane through (-17.2445, 0, 14.6352) normal (0, 0, 1) x (1, 0, 0)
  line L0 (29.283, 0) -> (29.283, 3.066)
  line L1 (29.283, 3.066) -> (31.7849, 3.066)
  line L2 (31.7849, 3.066) -> (31.7849, 0)
  line L3 (31.7849, 0) -> (29.283, 0)
  point P0 (17.2445, 0)
  dimension "d96" = 3.066
  dimension "d97" = 2.5019
  dimension "d98" = 12.0385
  constraints: 8 end point, 2 midpoint, 1 parallel, 1 perpendicular, 1 vertical
  measures "d96" distance of L0.start L0.end
  measures "d97" distance of L0.end L1.end
  measures "d98" distance from line of L0 point (17.244, 0)
sketch "Sketch28" plane through (12.0385, -1.5706, 16.2057) normal (0, -1, 0) x (1, 0, 0)
  line L0 (2.5019, 0) -> (2.5019, 1.4954) projected
  line L1 (2.5019, 1.4954) -> (2.5019, 0.1562)
  line L2 (0, 0) -> (2.5019, 0) projected
  line L3 (2.5019, 0.1562) -> (-26.579, 0.1562)
  line L4 (-26.579, -1.5706) -> (-26.579, 1.4954) projected
  line L5 (-26.579, 1.4954) -> (-26.579, 0.1562)
  line L6 (-26.579, 1.4954) -> (-24.0771, 1.4954) projected
  line L7 (2.5019, 1.4954) -> (0, 1.4954) projected
  line L8 (-26.579, 1.4954) -> (2.5019, 1.4954)
  point P0 (-12.0385, -16.2057)
  dimension "d139" = 0.1562
  constraints: 8 end point, 2 horizontal, 2 point on line, 1 collinear
  measures "d139" distance from line of L2 L1.end
sketch "Sketch29" plane through (14.5404, 0, 17.7012) normal (0, 0.9961947, -0.0871557) x (-1, 0, 0)
  line L0 (0, -1.5249) -> (0, -1.471) projected
  line L1 (14.5404, 4.9288) -> (29.0809, 4.9288)
  line L2 (29.0809, -0.1369) -> (29.0809, -1.471) projected
  line L3 (29.0809, -1.5249) -> (29.0809, -1.471) projected
  line L4 (14.5404, -1.5249) -> (29.0809, -1.5249)
  line L5 (29.0809, -1.5249) -> (31.3415, -1.5249)
  line L6 (31.3415, -0.5277) -> (27.9019, -6.9707) projected
  line L7 (31.3415, -1.5249) -> (31.3415, 4.9288)
  line L8 (31.3415, 4.9288) -> (29.0809, 4.9288)
  line L9 (14.5404, 4.9288) -> (14.5404, -0.1369) construction
  line L10 (14.5404, 4.9288) -> (0, 4.9288)
  line L11 (0, -1.5249) -> (0, -1.471)
  line L12 (14.5404, -1.5249) -> (0, -1.5249)
  line L13 (0, -1.5249) -> (-2.2606, -1.5249)
  line L14 (-2.2606, -1.5249) -> (-2.2606, 4.9288)
  line L15 (-2.2606, 4.9288) -> (0, 4.9288)
  line L16 (0, -0.1369) -> (29.0809, -0.1369) projected
  line L17 (14.5404, -1.5249) -> (14.5404, -3.1924)
  point P0 (14.5404, -17.6338)
  dimension "d153" = 2.2606
  dimension "d154" = 6.4537
  dimension "d155" = 14.5404
  constraints: 26 end point, 3 symmetric about line, 2 horizontal, 2 midpoint, 2 perpendicular, 2 vertical, 1 collinear
  measures "d153" distance of L7.end L1.end
  measures "d154" distance between parallel lines of L5 L8
  measures "d155" distance of L1.start L1.end
sketch "Sketch30" plane through (-14.5404, 0.4296, 22.6112) normal (0, 0.0871557, 0.9961947) x (1, 0, 0)
  line L0 (-4.3656, 0.2423) -> (-5.0264, -0.3929)
  arc A0 (-5.0264, -0.3929) -> (-2.2606, -1.5706) centre (-2.2606, 2.2659) ccw
  arc A1 (-4.3656, 0.2423) -> (-2.6924, 0) centre (-2.6924, 5.8985) ccw
  arc A2 (31.7849, 0) -> (33.4465, 0.2423) centre (31.7849, 5.8184) ccw
  line L1 (33.4465, 0.2423) -> (34.1072, -0.3929)
  arc A3 (31.3415, -1.5604) -> (34.1072, -0.3929) centre (31.3513, 2.276) ccw
  line L2 (-2.2606, 0) -> (-2.2606, -1.5706) projected
  line L3 (-2.2606, 0) -> (-2.2606, -1.5706)
  line L4 (31.7849, 0) -> (31.3415, 0)
  line L5 (31.3415, 2.9552) -> (31.3415, -1.5604) projected
  line L6 (31.3415, -1.5604) -> (31.3415, 0)
  line L7 (-2.6924, 0) -> (-2.2606, 0)
  point P0 (-4.193, 21.3713)
  dimension "d164" = 0.4318
  dimension "d165" = 0.9165
  constraints: 12 end point, 8 point on circle, 4 centre point, 2 collinear, 2 horizontal, 1 point on line
  measures "d164" horizontal distance of L7.start L2.end
  measures "d165" distance of L0.start L0.end
sketch "Sketch31" plane through (-17.2328, 0.4296, 22.6112) normal (0, 0.0871557, 0.9961947) x (1, 0, 0)
  line L0 (17.2328, -1.5705) -> (34.0466, -1.5705)
  line L1 (17.2328, -1.5705) -> (17.2328, -1.1091) construction
  line L2 (17.2328, -1.1091) -> (32.7512, -1.1091)
  line L3 (34.0466, -1.5705) -> (0.4191, -1.5705)
  line L4 (17.2328, -1.1091) -> (1.7145, -1.1091)
  line L5 (17.2328, -1.5705) -> (0.4191, -1.5705)
  arc A0 (32.7512, -1.1091) -> (36.1389, 0.2423) centre (32.7512, 3.8127) ccw
  arc A1 (34.0466, -1.5705) -> (37.4284, 0.4782) centre (34.0339, 2.2659) ccw
  line L6 (36.1389, 0.2423) -> (37.11, 0.6459)
  arc A2 (36.7996, -0.3929) -> (37.8703, 2.2659) centre (34.0339, 2.2659) ccw
  line L7 (37.4284, 0.4782) -> (37.11, 0.6459)
  arc A3 (-1.6732, 0.2423) -> (1.7145, -1.1091) centre (1.7145, 3.8127) ccw
  line L8 (-1.6732, 0.2423) -> (-2.6443, 0.6459)
  arc A4 (-2.9627, 0.4782) -> (0.4191, -1.5705) centre (0.4318, 2.2659) ccw
  line L9 (-2.9627, 0.4782) -> (-2.6443, 0.6459)
  line L10 (29.2714, 0) -> (5.1943, 0) projected
  point P0 (-2.334, -0.3929)
  point P1 (17.2328, 0)
  dimension "d174" = 0.3598
  dimension "d175" = 1.8415
  dimension "d176" = 1.2954
  constraints: 20 end point, 11 point on circle, 8 symmetric about line, 5 centre point, 2 midpoint, 1 collinear, 1 concentric, 1 line through centre, 1 perpendicular, 1 tangent, 2 other
  measures "d174" distance of L7.start L6.end
  measures "d175" distance of L7.start A2.end
  measures "d176" horizontal distance of L2.end L0.end
sketch "Sketch32" plane through (-17.2328, 0.4296, 22.6112) normal (0, 0.0871557, 0.9961947) x (1, 0, 0)
  line L0 (12.8773, -0.3397) -> (23.4924, -0.3397)
  line L1 (23.4924, -0.3397) -> (23.4924, -1.0552)
  line L2 (23.4924, -1.0552) -> (12.8773, -1.0552)
  line L3 (12.8773, -1.0552) -> (12.8773, -0.3397)
  line L4 (0, 0) -> (34.4773, 0) projected
  line L5 (17.2387, 0) -> (17.2387, -1.2858)
  point P0 (17.2328, 1.5428)
  point P1 (17.2387, -0.3397)
  dimension "d179" = 10.6151
  dimension "d180" = 0.7154
  dimension "d181" = 4.3614
  dimension "d182" = 0.3397
  constraints: 10 end point, 2 parallel, 2 perpendicular, 2 point on line, 1 horizontal, 1 midpoint, 1 vertical
  measures "d179" distance of L0.start L0.end
  measures "d180" distance of L0.end L1.end
  measures "d181" distance from line of L3 point (17.239, -0.34)
  measures "d182" distance between parallel lines of L0 L4
sketch "Sketch33" plane through (-17.2328, 0.0366, 18.1199) normal (0, 0.0871557, 0.9961947) x (1, 0, 0)
  line L0 (12.9302, -0.3926) -> (17.4387, -0.3926)
  line L1 (17.4387, -0.3926) -> (17.4387, -1.0022)
  line L2 (17.4387, -1.0022) -> (12.9302, -1.0022)
  line L3 (12.9302, -1.0022) -> (12.9302, -0.3926)
  line L4 (12.9302, -0.6974) -> (12.8773, -0.6974)
  line L5 (12.8773, -1.0552) -> (12.8773, -0.3397) projected
  line L6 (23.4924, -1.0552) -> (12.8773, -1.0552) projected
  line L7 (12.8773, -1.0552) -> (12.8773, -0.3397) projected
  line L8 (15.1844, -0.3926) -> (15.1844, -0.3397)
  point P0 (17.2328, 1.5428)
  dimension "d186" = 4.5085
  dimension "d187" = 0.6096
  dimension "d188" = 0.0529
  constraints: 12 end point, 3 midpoint, 3 perpendicular, 2 parallel, 1 horizontal, 1 vertical
  measures "d186" distance of L0.start L0.end
  measures "d187" distance of L0.end L1.end
  measures "d188" distance of L8.start L8.end
sketch "Sketch34" plane through (-17.2328, 0.0168, 17.8932) normal (0, 0.0871557, 0.9961947) x (1, 0, 0)
  line L0 (12.8773, -0.3397) -> (23.4924, -0.3397) projected
  line L1 (12.8773, -0.3397) -> (8.3159, -0.3397)
  line L2 (8.3159, -0.3397) -> (8.3159, -1.0552)
  line L3 (8.3159, -1.0552) -> (12.8773, -1.0552)
  line L4 (12.8773, -1.0552) -> (12.8773, -0.3397)
  point P0 (17.2328, 1.5428)
  dimension "d191" = 4.5614
  constraints: 8 end point, 2 parallel, 1 horizontal, 1 perpendicular
  measures "d191" distance between parallel lines of L4 L2
equation "\"d5\" = d3"
equation "\"d13\" = 0.5 * d3"
equation "\"d22\" = 0.666667 * d3"
body "Solid1"
